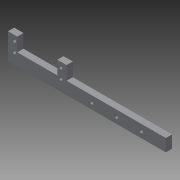
# Autodesk Inventor part: flapperservomount
Saved by Autodesk Inventor 2015 (Build 190159000, 159)
## iProperties
Created: 2015-02-15
Part Number: flapperservomount
Material: Generic
Document SubType Name: Modeling
Designer: sauhaarda
Density: 1 g/cm^3
Appearance: Default
Author: sauhaarda
Autodesk Inventor part; units mm, degrees
ref_plane "YZ Plane" through (0, 0, 0) normal (1, 0, 0) x (0, 1, 0)
ref_plane "XZ Plane" through (0, 0, 0) normal (0, 1, 0) x (-1, 0, 0)
ref_plane "XY Plane" through (0, 0, 0) normal (0, 0, 1) x (1, 0, 0)
sketch "Sketch1" plane through (0, 0, 0) normal (0, 0, 1) x (1, 0, 0)
  line L0 (101.6, 0) -> (101.6, -12.7)
  line L1 (101.6, -12.7) -> (0, -12.7)
  line L2 (50.8, 0) -> (0, 0)
  line L3 (50.8, 0) -> (101.6, 0)
  line L4 (0, -12.7) -> (50.8, -12.7)
  line L5 (50.8, -12.7) -> (101.6, -12.7)
  circle A0 centre (25.4, -6.35) radius 1.85
  circle A1 centre (50.8, -6.35) radius 1.85
  circle A2 centre (76.2, -6.35) radius 1.85
  line L6 (0, -12.7) -> (-60, -12.7)
  line L7 (-60, -12.7) -> (-60, 0)
  line L8 (-9.5, 0) -> (-9.5, 13.9)
  line L9 (-9.5, 13.9) -> (0, 13.9)
  line L10 (0, 13.9) -> (0, 0)
  line L11 (-50.5004, 13.8938) -> (-60, 13.8938)
  line L12 (-60, 13.8938) -> (-60, 0)
  line L13 (-50.5004, 13.8938) -> (-53.7504, 13.8938)
  circle A3 centre (-53.7504, 8.8938) radius 1.8542
  line L14 (-9.5, 13.9) -> (-6.2488, 13.9)
  line L15 (-9.5, 8.8962) -> (-9.5, 13.9)
  circle A4 centre (-6.2488, 8.8962) radius 1.8542
  line L16 (-53.7504, 13.8938) -> (-50.5004, 13.8938)
  circle A5 centre (-53.7504, -1.1062) radius 1.8542
  circle A6 centre (-6.2488, -1.1) radius 1.8542
  line L17 (-9.5, 0) -> (-50.5004, 0)
  line L18 (-50.5004, 13.8938) -> (-50.5004, 0)
  line L19 (0, 0) -> (0, -12.7)
  line L20 (0, 0) -> (101.6, 0)
  line L21 (101.6, 0) -> (101.6, -12.7)
  line L22 (101.6, -12.7) -> (0, -12.7)
  line L23 (-60, 13.8938) -> (-60, -12.7)
  line L24 (-60, -12.7) -> (0, -12.7)
  line L25 (0, -12.7) -> (0, 13.9)
  line L26 (0, 13.9) -> (-9.5, 13.9)
  line L27 (-9.5, 0) -> (-50.5004, 0)
  line L28 (-50.5004, 13.8938) -> (-60, 13.8938)
  dimension "d0" = 101.6
  dimension "d1" = 12.7
  dimension "d2" = 3.7
  dimension "d3" = 3.7
  dimension "d4" = 3.7
  dimension "d5" = 60
  dimension "d6" = 9.5
  dimension "d7" = 13.9
  dimension "d8" = 9.4996
  dimension "d9" = 13.8938
  dimension "d12" = 3.7084
  dimension "d15" = 3.7084
  dimension "d17" = 3.7084
  dimension "d19" = 3.7084
  constraints: 58 end point, 8 collinear, 7 centre point, 6 perpendicular, 4 horizontal, 1 midpoint, 1 parallel, 1 vertical
  measures "d0" distance of L0.end L1.end
  measures "d1" distance of L0.start L0.end
  measures "d2" diameter of A0
  measures "d3" diameter of A1
  measures "d4" diameter of A2
  measures "d5" distance of L7.end L10.end
  measures "d6" distance of L8.end L9.end
  measures "d7" distance of L8.start L8.end
  measures "d8" distance of L11.end L11.start
  measures "d9" distance of L11.start L17.end
  measures "d12" diameter of A3
  measures "d15" diameter of A4
  measures "d17" diameter of A5
  measures "d19" diameter of A6
extrude "Extrusion1" add sketch "Sketch1" along normal blind 6.35
body "Solid1"
